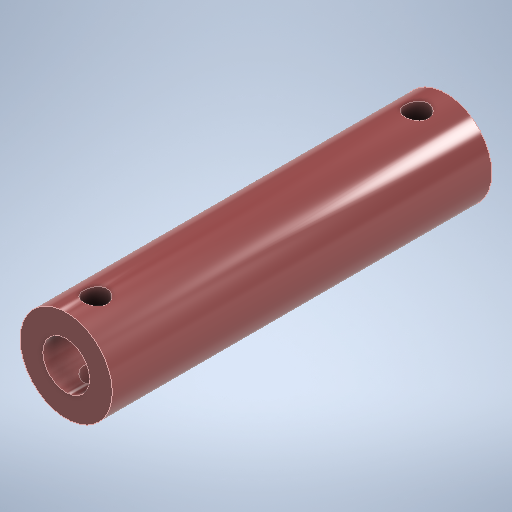
# Autodesk Inventor part: tube vers roue libre
Saved by Autodesk Inventor 2026.2 (Build 302298010, 298A)
## iProperties
Created: 2026-03-20
Part Number: tube vers roue libre
Material: Générique
Document SubType Name: Modeling
Designer: Genon
Density: 1 g/cm^3
Appearance: Châtaignier
Author: Genon
Autodesk Inventor part; units mm, degrees
ref_plane "YZ Plane" through (0, 0, 0) normal (1, 0, 0) x (0, 1, 0)
ref_plane "XZ Plane" through (0, 0, 0) normal (0, 1, 0) x (-1, 0, 0)
ref_plane "XY Plane" through (0, 0, 0) normal (0, 0, 1) x (1, 0, 0)
sketch "Esquisse1" plane through (0, 0, 0) normal (0, 0, 1) x (1, 0, 0)
  circle A0 centre (0, 0) radius 7.9
  circle A1 centre (0, 0) radius 4
  dimension "d0" = 15.8
  dimension "d1" = 8
  constraints: 2 centre point, 2 coincident
  measures "d0" diameter of A0
  measures "d1" diameter of A1
extrude "Extrusion1" add sketch "Esquisse1" along normal blind 65
sketch "Esquisse2" plane through (0, 0, 0) normal (0, 1, 0) x (-1, 0, 0)
  line L0 (7.9, 65) -> (-7.9, 65) projected
  line L1 (0, 65) -> (0, 60)
  line L2 (0, 0) -> (0, 5)
  dimension "d4" = 5
  dimension "d5" = 5
  constraints: 4 end point, 2 coincident, 2 vertical, 1 midpoint
  measures "d4" distance of L1.start L1.end
  measures "d5" distance of L2.start L2.end
hole "Perçage1" at (0, 0, 60) at (0, 0, 5) direction (0, -1, 0) diameter 4 end through all both
